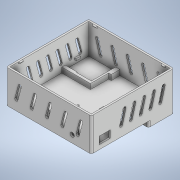
# Autodesk Inventor part: Raspberry Pi hållare 2
Saved by Autodesk Inventor 2021 (Build 250183000, 183)
## iProperties
Created: 2024-12-11
Part Number: Raspberry Pi hållare 2
Material: Generic
Document SubType Name: Modeling
Designer: 22liatho
Density: 1 g/cm^3
Appearance: Default
Author: 22liatho
Autodesk Inventor part; units mm, degrees
ref_plane "YZ Plane" through (0, 0, 0) normal (1, 0, 0) x (0, 1, 0)
ref_plane "XZ Plane" through (0, 0, 0) normal (0, 1, 0) x (-1, 0, 0)
ref_plane "XY Plane" through (0, 0, 0) normal (0, 0, 1) x (1, 0, 0)
sketch "Sketch1" plane through (0, 0, 0) normal (0, 1, 0) x (-1, 0, 0)
  line L0 (0, 0) -> (-94.1, 0)
  line L1 (-94.1, 0) -> (-94.1, -91.1)
  line L2 (-94.1, -91.1) -> (0, -91.1)
  line L3 (0, -91.1) -> (0, 0)
  line L4 (2, 2) -> (-96.1, 2)
  line L5 (-96.1, 2) -> (-96.1, -93.1)
  line L6 (-96.1, -93.1) -> (2, -93.1)
  line L7 (2, -93.1) -> (2, 2)
  dimension "d0" = 91.1
  dimension "d1" = 94.1
  dimension "d2" = 2
  dimension "d3" = 2
  dimension "d4" = 2
  dimension "d5" = 2
  constraints: 16 end point, 4 parallel, 2 horizontal, 2 perpendicular
  measures "d0" distance of L2.end L0.start
  measures "d1" distance of L1.end L2.end
  measures "d2" distance between parallel lines of L6 L2
  measures "d3" distance between parallel lines of L7 L3
  measures "d4" distance between parallel lines of L4 L0
  measures "d5" distance between parallel lines of L1 L5
extrude "Extrusion1" add sketch "Sketch1" along normal blind 2 contours L3 L2 L1 L0
extrude "Extrusion2" add sketch "Sketch1" along normal blind 38.2
sketch "Sketch3" plane through (96.1, 0, 2) normal (1, 0, 0) x (0, 0, -1)
  line L0 (12.85, 3.6) -> (19.55, 3.6)
  line L1 (19.55, 6.8) -> (12.85, 6.8)
  line L2 (11.7, 5.65) -> (11.7, 4.75)
  line L3 (20.7, 4.75) -> (20.7, 5.65)
  arc A0 (12.85, 6.8) -> (11.7, 5.65) centre (12.85, 5.65) ccw
  arc A1 (11.7, 4.75) -> (12.85, 3.6) centre (12.85, 4.75) ccw
  arc A2 (20.7, 5.65) -> (19.55, 6.8) centre (19.55, 5.65) ccw
  arc A3 (19.55, 3.6) -> (20.7, 4.75) centre (19.55, 4.75) ccw
  line L4 (0, 0) -> (0, 38.2) projected
  line L5 (0, 0) -> (95.1, 0) projected
  line L6 (12.85, 8.4) -> (19.55, 8.4)
  arc A4 (22.3, 5.65) -> (19.55, 8.4) centre (19.55, 5.65) ccw
  line L7 (22.3, 5.65) -> (22.3, 4.75)
  arc A5 (19.55, 2) -> (22.3, 4.75) centre (19.55, 4.75) ccw
  line L8 (19.55, 2) -> (12.85, 2)
  arc A6 (10.1, 4.75) -> (12.85, 2) centre (12.85, 4.75) ccw
  line L9 (10.1, 4.75) -> (10.1, 5.65)
  arc A7 (12.85, 8.4) -> (10.1, 5.65) centre (12.85, 5.65) ccw
  point P0 (2, 0)
  dimension "d15" = 1.15
  dimension "d16" = 9
  dimension "d17" = 3.2
  dimension "d18" = 11.7
  dimension "d19" = 3.6
  dimension "d22" = 1.6
  constraints: 16 end point, 16 point on circle, 8 centre point, 8 tangent, 3 equal radius, 2 horizontal, 2 perpendicular, 1 vertical, 7 other
  measures "d15" radius of A0
  measures "d16" distance between parallel lines of L2 L3
  measures "d17" distance between parallel lines of L1 L0
  measures "d18" distance between parallel lines of L4 L2
  measures "d19" distance between parallel lines of L5 L0
  measures "d22" distance between parallel lines of L1 L6
sketch "Sketch4" plane through (0, 0, 0) normal (0, -1, 0) x (1, 0, 0)
  line L0 (96.1, 2) -> (96.1, -93.1) projected
  line L1 (96.1, -93.1) -> (91.1, -93.1)
  line L2 (91.1, -93.1) -> (91.1, -68.8)
  line L3 (66.1, -63.8) -> (96.1, -63.8)
  line L4 (96.1, -63.8) -> (96.1, -93.1)
  line L5 (96.1, -93.1) -> (-2, -93.1) projected
  line L6 (71.1, -93.1) -> (66.1, -93.1)
  line L7 (66.1, -93.1) -> (66.1, -63.8)
  line L8 (71.1, -68.8) -> (71.1, -93.1)
  line L9 (71.1, -68.8) -> (91.1, -68.8)
  line L10 (93.1, -93.1) -> (93.1, -66.8)
  line L11 (93.1, -66.8) -> (69.1, -66.8)
  line L12 (69.1, -66.8) -> (69.1, -93.1)
  point P0 (0, 0)
  point P1 (96.1, -63.8)
  point P2 (66.1, -93.1)
  dimension "d25" = 5
  dimension "d26" = 5
  dimension "d28" = 26.3
  dimension "d29" = 24
  dimension "d30" = 2
  dimension "d31" = 2
  dimension "d32" = 2
  dimension "d33" = 5
  constraints: 22 end point, 4 parallel, 4 perpendicular, 3 point on line, 2 horizontal
  measures "d25" distance between parallel lines of L0 L2
  measures "d26" distance between parallel lines of L7 L8
  measures "d28" distance of L11.end L12.end
  measures "d29" distance between parallel lines of L12 L10
  measures "d30" distance between parallel lines of L12 L8
  measures "d31" distance between parallel lines of L11 L9
  measures "d32" distance between parallel lines of L10 L2
  measures "d33" distance between parallel lines of L9 L3
extrude "Extrusion6" add sketch "Sketch4" along normal blind 6.5 contours L0 L1 L10 L11 L12 L5 L7 L3 | L1 L2 L9 L8 L5 L12 L11 L10
sketch "Sketch5" plane through (96.1, 38.2, -93.1) normal (0, 0, -1) x (-1, 0, 0)
  line L0 (98.1, -38.2) -> (0, -38.2) projected
  line L1 (2.5, -38.2) -> (27.5, -38.2)
  line L2 (27.5, -38.2) -> (27.5, -43.2)
  line L3 (27.5, -43.2) -> (2.5, -43.2)
  line L4 (2.5, -43.2) -> (2.5, -38.2)
  line L5 (25, -38.2) -> (25, -44.7) projected
  line L6 (5, -38.2) -> (5, -44.7) projected
  line L7 (25, -44.7) -> (5, -44.7) projected
  point P0 (96.1, -38.2)
  dimension "d37" = 2.5
  dimension "d38" = 2.5
  dimension "d418" = 1.5
  constraints: 8 end point, 2 parallel, 1 horizontal, 1 perpendicular, 1 point on line
  measures "d37" distance between parallel lines of L5 L2
  measures "d38" distance between parallel lines of L6 L4
  measures "d418" distance between parallel lines of L7 L3
extrude "Extrusion7" cut sketch "Sketch5" against normal up to surface (24.3 mm away) contours L2 L3 L5 L0 | L5 L3 L6 L0 | L6 L3 L4 L0
sketch "Sketch6" plane through (0, 0, 0) normal (0, -1, 0) x (1, 0, 0)
  line L0 (58.6, -6.3) -> (7.5, -6.3)
  arc A0 (7.5, -6.3) -> (7.5, -9.8) centre (7.5, -8.05) ccw
  line L1 (7.5, -9.8) -> (58.6, -9.8)
  arc A1 (58.6, -9.8) -> (58.6, -6.3) centre (58.6, -8.05) ccw
  line L2 (96.1, 2) -> (96.1, -63.8) projected
  line L3 (0, 0) -> (94.1, 0) projected
  line L4 (58.6, -18.5167) -> (7.5, -18.5167)
  line L5 (7.5, -22.0167) -> (58.6, -22.0167)
  arc A2 (7.5, -18.5167) -> (7.5, -22.0167) centre (7.5, -20.2667) ccw
  arc A3 (58.6, -22.0167) -> (58.6, -18.5167) centre (58.6, -20.2667) ccw
  line L6 (58.6, -30.7333) -> (7.5, -30.7333)
  line L7 (7.5, -34.2333) -> (58.6, -34.2333)
  arc A4 (7.5, -30.7333) -> (7.5, -34.2333) centre (7.5, -32.4833) ccw
  arc A5 (58.6, -34.2333) -> (58.6, -30.7333) centre (58.6, -32.4833) ccw
  line L8 (58.6, -42.95) -> (7.5, -42.95)
  line L9 (7.5, -46.45) -> (58.6, -46.45)
  arc A6 (7.5, -42.95) -> (7.5, -46.45) centre (7.5, -44.7) ccw
  arc A7 (58.6, -46.45) -> (58.6, -42.95) centre (58.6, -44.7) ccw
  line L10 (58.6, -55.1667) -> (7.5, -55.1667)
  line L11 (7.5, -58.6667) -> (58.6, -58.6667)
  arc A8 (7.5, -55.1667) -> (7.5, -58.6667) centre (7.5, -56.9167) ccw
  arc A9 (58.6, -58.6667) -> (58.6, -55.1667) centre (58.6, -56.9167) ccw
  line L12 (58.6, -67.3833) -> (7.5, -67.3833)
  line L13 (7.5, -70.8833) -> (58.6, -70.8833)
  arc A10 (7.5, -67.3833) -> (7.5, -70.8833) centre (7.5, -69.1333) ccw
  arc A11 (58.6, -70.8833) -> (58.6, -67.3833) centre (58.6, -69.1333) ccw
  line L14 (58.6, -79.6) -> (7.5, -79.6)
  line L15 (7.5, -83.1) -> (58.6, -83.1)
  arc A12 (7.5, -79.6) -> (7.5, -83.1) centre (7.5, -81.35) ccw
  arc A13 (58.6, -83.1) -> (58.6, -79.6) centre (58.6, -81.35) ccw
  line L16 (66.1, -93.1) -> (-2, -93.1) projected
  line L17 (66.1, -63.8) -> (66.1, -93.1) projected
  arc A14 (106.65, -9.8) -> (106.65, -6.3) centre (106.65, -8.05) ccw
  line L18 (106.65, -6.3) -> (55.55, -6.3)
  line L19 (55.55, -9.8) -> (106.65, -9.8)
  arc A15 (55.55, -6.3) -> (55.55, -9.8) centre (55.55, -8.05) ccw
  line L20 (55.55, -22.3) -> (106.65, -22.3)
  arc A16 (106.65, -22.3) -> (106.65, -18.8) centre (106.65, -20.55) ccw
  line L21 (106.65, -18.8) -> (55.55, -18.8)
  arc A17 (55.55, -18.8) -> (55.55, -22.3) centre (55.55, -20.55) ccw
  line L22 (55.55, -34.8) -> (106.65, -34.8)
  arc A18 (106.65, -34.8) -> (106.65, -31.3) centre (106.65, -33.05) ccw
  line L23 (106.65, -31.3) -> (55.55, -31.3)
  arc A19 (55.55, -31.3) -> (55.55, -34.8) centre (55.55, -33.05) ccw
  line L24 (55.55, -47.3) -> (106.65, -47.3)
  arc A20 (106.65, -47.3) -> (106.65, -43.8) centre (106.65, -45.55) ccw
  line L25 (106.65, -43.8) -> (55.55, -43.8)
  arc A21 (55.55, -43.8) -> (55.55, -47.3) centre (55.55, -45.55) ccw
  line L26 (55.55, -59.8) -> (106.65, -59.8)
  arc A22 (106.65, -59.8) -> (106.65, -56.3) centre (106.65, -58.05) ccw
  line L27 (106.65, -56.3) -> (55.55, -56.3)
  arc A23 (55.55, -56.3) -> (55.55, -59.8) centre (55.55, -58.05) ccw
  line L28 (55.55, -72.3) -> (106.65, -72.3)
  arc A24 (106.65, -72.3) -> (106.65, -68.8) centre (106.65, -70.55) ccw
  line L29 (106.65, -68.8) -> (55.55, -68.8)
  arc A25 (55.55, -68.8) -> (55.55, -72.3) centre (55.55, -70.55) ccw
  line L30 (55.55, -84.8) -> (106.65, -84.8)
  arc A26 (106.65, -84.8) -> (106.65, -81.3) centre (106.65, -83.05) ccw
  line L31 (106.65, -81.3) -> (55.55, -81.3)
  arc A27 (55.55, -81.3) -> (55.55, -84.8) centre (55.55, -83.05) ccw
  line L32 (71.1, -68.8) -> (91.1, -68.8) projected
  line L33 (91.1, -68.8) -> (91.1, -93.1) projected
  line L34 (71.1, -93.1) -> (71.1, -68.8) projected
  line L35 (96.1, -63.8) -> (66.1, -63.8) projected
  line L36 (91.1, -93.1) -> (-2, -93.1) projected
  line L37 (-2, 2) -> (96.1, 2) projected
  point P0 (93.6, -93.1)
  point P1 (68.6, -93.1)
  point P2 (96.1, -93.1)
  dimension "d42" = 7.5
  dimension "d43" = 3.5
  dimension "d47" = 12.2167
  dimension "d52" = 10
  dimension "d53" = 7.5
  dimension "d56" = 48.05
  dimension "d64" = 12.5
  dimension "d70" = 15.55
  dimension "d71" = 15.55
  dimension "d74" = 8.3
  dimension "d75" = 8.3
  constraints: 56 end point, 56 point on circle, 28 centre point, 4 tangent, 3 horizontal, 2 vertical, 1 point on line, 130 other
  measures "d42" horizontal distance of L3.start L1.start
  measures "d43" distance between parallel lines of L1 L0
  measures "d47" distance of L0.start L4.start
  measures "d52" distance between parallel lines of L16 L15
  measures "d53" distance from line of A13.centre L17
  measures "d56" distance of A1.centre A14.centre
  measures "d64" distance of L19.start L20.start
  measures "d70" distance from line of L33 A24.centre
  measures "d71" distance from line of L34 A27.centre
  measures "d74" distance between parallel lines of L37 L18
  measures "d75" distance between parallel lines of L36 L30
sketch "Sketch7" plane through (0, 0, 0) normal (0, -1, 0) x (1, 0, 0)
  line L0 (83.6, -43.799) -> (10.5, -43.799)
  arc A0 (83.6, -47.299) -> (83.6, -43.799) centre (83.6, -45.549) ccw
  line L1 (83.6, -47.299) -> (10.5, -47.299)
  arc A1 (10.5, -43.799) -> (10.5, -47.299) centre (10.5, -45.549) ccw
  line L2 (96.1, 2) -> (96.1, -63.8) projected
  line L3 (91.1, -68.8) -> (91.1, -93.1) projected
  line L4 (71.1, -93.1) -> (71.1, -68.8) projected
  line L5 (-2, -93.1) -> (-2, 2) projected
  line L6 (83.6, -59.2327) -> (10.5, -59.2327)
  arc A2 (10.5, -55.7327) -> (10.5, -59.2327) centre (10.5, -57.4827) ccw
  line L7 (83.6, -55.7327) -> (10.5, -55.7327)
  arc A3 (83.6, -59.2327) -> (83.6, -55.7327) centre (83.6, -57.4827) ccw
  line L8 (56.1, -67.6663) -> (10.5, -67.6663)
  arc A4 (10.5, -67.6663) -> (10.5, -71.1663) centre (10.5, -69.4163) ccw
  line L9 (10.5, -71.1663) -> (56.1, -71.1663)
  arc A5 (56.1, -71.1663) -> (56.1, -67.6663) centre (56.1, -69.4163) ccw
  line L10 (-2, 2) -> (96.1, 2) projected
  line L11 (96.1, -63.8) -> (66.1, -63.8) projected
  line L12 (66.1, -63.8) -> (66.1, -93.1) projected
  line L13 (10.5, -83.1) -> (56.1, -83.1)
  arc A6 (10.5, -79.6) -> (10.5, -83.1) centre (10.5, -81.35) ccw
  line L14 (56.1, -79.6) -> (10.5, -79.6)
  arc A7 (56.1, -83.1) -> (56.1, -79.6) centre (56.1, -81.35) ccw
  line L15 (66.1, -93.1) -> (-2, -93.1) projected
  line L16 (83.6, -19.9317) -> (38, -19.9317)
  arc A8 (38, -19.9317) -> (38, -23.4317) centre (38, -21.6817) ccw
  line L17 (38, -23.4317) -> (83.6, -23.4317)
  arc A9 (83.6, -23.4317) -> (83.6, -19.9317) centre (83.6, -21.6817) ccw
  arc A10 (38, -7.9977) -> (38, -11.4977) centre (38, -9.7477) ccw
  line L18 (38, -11.4977) -> (83.6, -11.4977)
  arc A11 (83.6, -11.4977) -> (83.6, -7.9977) centre (83.6, -9.7477) ccw
  line L19 (83.6, -7.9977) -> (38, -7.9977)
  line L20 (83.6, -31.8653) -> (10.5, -31.8653)
  arc A12 (83.6, -35.3653) -> (83.6, -31.8653) centre (83.6, -33.6153) ccw
  arc A13 (10.5, -31.8653) -> (10.5, -35.3653) centre (10.5, -33.6153) ccw
  line L21 (83.6, -35.3653) -> (10.5, -35.3653)
  point P0 (0, 0)
  point P1 (96.1, -93.1)
  dimension "d76" = 3.5
  dimension "d80" = 12.5
  dimension "d81" = 12.5
  dimension "d84" = 11.9337
  dimension "d89" = 45.799
  dimension "d92" = 10
  dimension "d93" = 3.5
  dimension "d96" = 11.9337
  dimension "d102" = 10
  dimension "d391" = 11.9337
  dimension "d392" = 12.5
  dimension "d393" = 3.5
  dimension "d394" = 12.5
  dimension "d395" = 45.6
  dimension "d396" = 45.6
  dimension "d397" = 23.8673
  dimension "d400" = 11.934
  dimension "d411" = 11.9337
  constraints: 28 end point, 28 point on circle, 14 centre point, 12 tangent, 6 horizontal, 4 vertical, 40 other
  measures "d76" distance between parallel lines of L0 L1
  measures "d80" distance from line of L5 A1.centre
  measures "d81" distance from line of L2 A0.centre
  measures "d84" distance of L1.start L6.start
  measures "d89" distance between parallel lines of L10 L0
  measures "d92" distance from line of L12 A5.centre
  measures "d93" distance between parallel lines of L9 L8
  measures "d96" distance of L9.start L13.start
  measures "d102" distance between parallel lines of L15 L13
  measures "d391" distance between parallel lines of L9 L6
  measures "d392" distance from line of L5 A6.centre
  measures "d393" distance between parallel lines of L17 L16
  measures "d394" distance from line of L2 A9.centre
  measures "d395" distance of L8.start L8.end
  measures "d396" distance of L16.start L16.end
  measures "d397" distance between parallel lines of L0 L16
  measures "d400" distance of L17.start L18.start
  measures "d411" distance of L0.start L20.start
extrude "Extrusion8" [suppressed]
sketch "Sketch10" plane through (-2, 0, 2) normal (0, 0, 1) x (1, 0, 0)
  arc A0 (17.4, 26.1471) -> (14.0192, 27.0529) centre (15.7096, 26.6) ccw
  arc A1 (10, 12.0529) -> (13.3807, 11.1471) centre (11.6904, 11.6) ccw
  line L0 (13.3807, 11.1471) -> (17.4, 26.1471)
  line L1 (10, 12.0529) -> (14.0192, 27.0529)
  line L2 (0, 38.2) -> (98.1, 38.2)
  line L3 (13.3807, 11.1471) -> (14.3807, 11.1471)
  line L4 (14.3807, 11.1471) -> (13.8807, 11.1471)
  line L5 (98.1, 0) -> (98.1, 38.2) projected
  line L6 (0, 0) -> (98.1, 0) projected
  line L7 (0, 0) -> (0, 38.2) projected
  arc A2 (27.675, 12.0529) -> (31.0557, 11.1471) centre (29.3654, 11.6) ccw
  line L8 (27.675, 12.0529) -> (31.6942, 27.0529)
  line L9 (32.0557, 11.1471) -> (31.5557, 11.1471)
  line L10 (31.0557, 11.1471) -> (35.075, 26.1471)
  arc A3 (35.075, 26.1471) -> (31.6942, 27.0529) centre (33.3846, 26.6) ccw
  line L11 (31.0557, 11.1471) -> (32.0557, 11.1471)
  arc A4 (45.35, 12.0529) -> (48.7308, 11.1471) centre (47.0404, 11.6) ccw
  line L12 (45.35, 12.0529) -> (49.3692, 27.0529)
  line L13 (49.7308, 11.1471) -> (49.2308, 11.1471)
  line L14 (48.7308, 11.1471) -> (52.75, 26.1471)
  arc A5 (52.75, 26.1471) -> (49.3692, 27.0529) centre (51.0596, 26.6) ccw
  line L15 (48.7308, 11.1471) -> (49.7308, 11.1471)
  arc A6 (63.025, 12.0529) -> (66.4058, 11.1471) centre (64.7154, 11.6) ccw
  line L16 (63.025, 12.0529) -> (67.0443, 27.0529)
  line L17 (67.4058, 11.1471) -> (66.9058, 11.1471)
  line L18 (66.4058, 11.1471) -> (70.425, 26.1471)
  arc A7 (70.425, 26.1471) -> (67.0443, 27.0529) centre (68.7346, 26.6) ccw
  line L19 (66.4058, 11.1471) -> (67.4058, 11.1471)
  arc A8 (80.7, 12.0529) -> (84.0808, 11.1471) centre (82.3904, 11.6) ccw
  line L20 (80.7, 12.0529) -> (84.7193, 27.0529)
  line L21 (85.0808, 11.1471) -> (84.5808, 11.1471)
  line L22 (84.0808, 11.1471) -> (88.1, 26.1471)
  arc A9 (88.1, 26.1471) -> (84.7193, 27.0529) centre (86.4096, 26.6) ccw
  line L23 (84.0808, 11.1471) -> (85.0808, 11.1471)
  dimension "d133" = 3.5
  dimension "d134" = 15
  dimension "d137" = 75
  dimension "d138" = 1
  dimension "d145" = 10
  dimension "d364" = 11.6
  dimension "d365" = 11.6
  dimension "d368" = 17.675
  dimension "d376" = 10
  constraints: 42 end point, 20 point on circle, 10 centre point, 4 tangent, 3 horizontal, 1 midpoint, 1 parallel, 56 other
  measures "d133" distance between parallel lines of L1 L0
  measures "d134" vertical distance of A1.centre A0.centre
  measures "d137" angle of L0 L3
  measures "d138" distance of L0.start L4.start
  measures "d145" distance from line of L7 L1.start
  measures "d364" distance from line of L6 A1.centre
  measures "d365" distance from line of L2 A0.centre
  measures "d368" distance of L1.start L8.start
  measures "d376" distance from line of L5 L22.end
sketch "Sketch9" plane through (-2, 0, 2) normal (0, 0, 1) x (1, 0, 0)
  line L0 (73.6, 6) -> (78.6, 6)
  line L1 (78.6, 6) -> (78.6, 11)
  line L2 (78.6, 11) -> (73.6, 11)
  line L3 (73.6, 11) -> (73.6, 6)
  line L4 (0, 0) -> (98.1, 0) projected
  line L5 (98.1, 0) -> (98.1, 38.2) projected
  circle A0 centre (76.1, 8.5) radius 2.5
  point P0 (2, 0)
  dimension "d126" = 5
  dimension "d127" = 19.5
  dimension "d128" = 5
  dimension "d380" = 5
  dimension "d475" = 8.5
  constraints: 8 end point, 2 parallel, 2 tangent, 1 centre point, 1 horizontal, 1 perpendicular
  measures "d126" distance between parallel lines of L3 L1
  measures "d127" distance between parallel lines of L5 L1
  measures "d128" distance between parallel lines of L0 L2
  measures "d380" diameter of A0
  measures "d475" distance from line of L4 A0.centre
extrude "Extrusion10" cut sketch "Sketch10" against normal blind 10 contours L0 A1 L1 A0
sketch "Sketch12" plane through (0, 2, -91.1) normal (0, 0, 1) x (1, 0, 0)
  line L0 (96.1, 36.2) -> (-2, 36.2) projected
  line L1 (5, 36.2) -> (10, 36.2)
  line L2 (10, 36.2) -> (10, 34.2)
  line L3 (10, 34.2) -> (5, 34.2)
  line L4 (5, 34.2) -> (5, 36.2)
  line L5 (84.1, 36.2) -> (89.1, 36.2)
  line L6 (89.1, 36.2) -> (89.1, 34.2)
  line L7 (89.1, 34.2) -> (84.1, 34.2)
  line L8 (84.1, 34.2) -> (84.1, 36.2)
  line L9 (0, 0) -> (0, 36.2) projected
  line L10 (94.1, 0) -> (94.1, 36.2) projected
  point P0 (0, -2)
  point P1 (-2, 36.2)
  point P2 (58.1, 29.2)
  dimension "d170" = 5
  dimension "d171" = 2
  dimension "d172" = 5
  dimension "d173" = 5
  dimension "d536" = 5
  constraints: 16 end point, 4 parallel, 2 horizontal, 2 perpendicular, 1 point on line, 3 other
  measures "d170" distance of L2.end L3.end
  measures "d171" distance of L1.end L2.end
  measures "d172" distance of L6.end L7.end
  measures "d173" distance between parallel lines of L9 L4
  measures "d536" distance from line of L10 L5.end
extrude "Extrusion11" add sketch "Sketch12" along normal blind 1.4
sketch "Sketch13" plane through (0, 2, -91.1) normal (1, 0, 0) x (0, 0, -1)
  line L0 (2, 36.2) -> (-93.1, 36.2) projected
  line L1 (-81.1, 36.2) -> (-76.1, 36.2)
  line L2 (-76.1, 36.2) -> (-76.1, 34.2)
  line L3 (-76.1, 34.2) -> (-81.1, 34.2)
  line L4 (-81.1, 34.2) -> (-81.1, 36.2)
  line L5 (-91.1, 0) -> (-91.1, 36.2) projected
  point P0 (-91.1, -2)
  point P1 (-76.1, 36.2)
  dimension "d201" = 2
  dimension "d202" = 5
  dimension "d203" = 10
  constraints: 8 end point, 2 parallel, 1 horizontal, 1 perpendicular, 1 point on line
  measures "d201" distance of L1.end L2.end
  measures "d202" distance of L2.end L3.end
  measures "d203" distance between parallel lines of L5 L4
extrude "Extrusion12" add sketch "Sketch13" along normal blind 1.4
chamfer "Chamfer9" distance 0.75 distance2 1.4 1 edges at (1.4, 38.2, -12.5) measured on face at (1.4, 37.5333, -11.6667)
chamfer "Chamfer10" distance 0.75 distance2 1.4 1 edges at (1.4, 36.825, -10) measured on face at (1.4, 37.0333, -11.6667)
chamfer "Chamfer11" distance 0.75 distance2 1.4 1 edges at (1.4, 36.825, -15) measured on face at (1.4, 37.0333, -12.1666)
chamfer "Chamfer12" distance 0.75 distance2 1.4 1 edges at (1.4, 36.2, -12.5) measured on face at (1.4, 37.0333, -11.9166)
sketch "Sketch14" plane through (94.1, 2, -91.1) normal (-1, 0, 0) x (0, 0, 1)
  line L0 (93.1, 36.2) -> (-2, 36.2) projected
  line L1 (81.1, 36.2) -> (76.1, 36.2)
  line L2 (76.1, 36.2) -> (76.1, 34.2)
  line L3 (76.1, 34.2) -> (81.1, 34.2)
  line L4 (81.1, 34.2) -> (81.1, 36.2)
  line L5 (93.1, -2) -> (93.1, 36.2) projected
  line L6 (91.1, 0) -> (91.1, 36.2) projected
  point P0 (91.1, -2)
  dimension "d242" = 5
  dimension "d243" = 2
  dimension "d537" = 10
  constraints: 8 end point, 2 parallel, 1 horizontal, 1 perpendicular, 1 point on line
  measures "d242" distance of L2.end L3.end
  measures "d243" distance of L3.end L1.start
  measures "d537" distance between parallel lines of L6 L4
extrude "Extrusion13" add sketch "Sketch14" along normal blind 1.4
chamfer "Chamfer25" distance 0.75 distance2 1.4 1 edges at (10, 37.2, -89.7) measured on face at (8.3333, 36.8667, -89.7)
chamfer "Chamfer26" distance 0.75 distance2 1.4 1 edges at (5, 37.2, -89.7) measured on face at (6.4167, 36.8667, -89.7)
chamfer "Chamfer27" distance 0.75 distance2 1.4 2 edges at (7.5, 38.2, -89.7) (86.6, 38.2, -89.7) measured on face at (87.4333, 36.8667, -89.7) measured on face at (6.9166, 36.8667, -89.7)
chamfer "Chamfer28" distance 0.75 distance2 1.4 1 edges at (7.5, 36.2, -89.7) measured on face at (6.9166, 36.6167, -89.7)
chamfer_without_effect "Chamfer29"
chamfer "Chamfer30" distance 0.75 distance2 1.4 1 edges at (84.1, 36.825, -89.7) measured on face at (85.7667, 37.0333, -89.7)
chamfer "Chamfer31" distance 0.75 distance2 1.4 1 edges at (86.9749, 36.2, -89.7) measured on face at (86.2666, 37.0333, -89.7)
chamfer "Chamfer32" distance 0.75 distance2 1.4 1 edges at (89.1, 37.2, -89.7) measured on face at (86.2666, 37.2833, -89.7)
chamfer "Chamfer33" distance 0.75 distance2 1.4 1 edges at (92.7, 37.2, -10) measured on face at (92.7, 36.8667, -11.6667)
chamfer "Chamfer34" distance 0.75 distance2 1.4 1 edges at (92.7, 37.2, -15) measured on face at (92.7, 36.8667, -12.1666)
chamfer "Chamfer35" distance 0.75 distance2 1.4 1 edges at (92.7, 38.2, -12.5) measured on face at (92.7, 36.8667, -11.9166)
chamfer "Chamfer36" distance 0.75 distance2 1.4 1 edges at (92.7, 36.2, -12.5) measured on face at (92.7, 36.6167, -11.9166)
sketch "Sketch16" plane through (96.1, 38.2, -93.1) normal (0, 0, -1) x (-1, 0, 0)
  line L0 (10, -26.6) -> (14.0192, -11.6)
  arc A0 (10, -26.6) -> (13.3807, -27.5059) centre (11.6904, -27.0529) ccw
  line L1 (14.3807, -27.5059) -> (13.8807, -27.5059)
  line L2 (13.3807, -27.5059) -> (17.4, -12.5059)
  line L3 (13.3807, -27.5059) -> (14.3807, -27.5059)
  arc A1 (17.4, -12.5059) -> (14.0192, -11.6) centre (15.7096, -12.0529) ccw
  line L4 (98.1, -38.2) -> (98.1, 0) projected
  line L5 (0, -44.7) -> (0, 0) projected
  line L6 (0, 0) -> (98.1, 0) projected
  arc A2 (27.675, -26.6) -> (31.0557, -27.5059) centre (29.3654, -27.0529) ccw
  line L7 (27.675, -26.6) -> (31.6942, -11.6)
  line L8 (32.0557, -27.5059) -> (31.5557, -27.5059)
  line L9 (31.0557, -27.5059) -> (32.0557, -27.5059)
  line L10 (31.0557, -27.5059) -> (35.075, -12.5059)
  arc A3 (35.075, -12.5059) -> (31.6942, -11.6) centre (33.3846, -12.0529) ccw
  arc A4 (45.35, -26.6) -> (48.7308, -27.5059) centre (47.0404, -27.0529) ccw
  line L11 (45.35, -26.6) -> (49.3692, -11.6)
  line L12 (49.7308, -27.5059) -> (49.2308, -27.5059)
  line L13 (48.7308, -27.5059) -> (49.7308, -27.5059)
  line L14 (48.7308, -27.5059) -> (52.75, -12.5059)
  arc A5 (52.75, -12.5059) -> (49.3692, -11.6) centre (51.0596, -12.0529) ccw
  arc A6 (63.025, -26.6) -> (66.4058, -27.5059) centre (64.7154, -27.0529) ccw
  line L15 (63.025, -26.6) -> (67.0443, -11.6)
  line L16 (67.4058, -27.5059) -> (66.9058, -27.5059)
  line L17 (66.4058, -27.5059) -> (67.4058, -27.5059)
  line L18 (66.4058, -27.5059) -> (70.425, -12.5059)
  arc A7 (70.425, -12.5059) -> (67.0443, -11.6) centre (68.7346, -12.0529) ccw
  arc A8 (80.7, -26.6) -> (84.0808, -27.5059) centre (82.3904, -27.0529) ccw
  line L19 (80.7, -26.6) -> (84.7193, -11.6)
  line L20 (85.0808, -27.5059) -> (84.5808, -27.5059)
  line L21 (84.0808, -27.5059) -> (85.0808, -27.5059)
  line L22 (84.0808, -27.5059) -> (88.1, -12.5059)
  arc A9 (88.1, -12.5059) -> (84.7193, -11.6) centre (86.4096, -12.0529) ccw
  point P0 (96.1, -38.2)
  point P1 (98.1, -19.1)
  point P2 (12.0096, -19.1)
  point P3 (29.6846, -19.1)
  point P4 (47.3596, -19.1)
  point P5 (65.0346, -19.1)
  point P6 (82.7096, -19.1)
  point P7 (98.1, -19.1)
  point P8 (0, -38.2)
  dimension "d327" = 3.5
  dimension "d328" = 15
  dimension "d329" = 75
  dimension "d330" = 1
  dimension "d336" = 17.675
  dimension "d377" = 10
  dimension "d378" = 10
  constraints: 40 end point, 20 point on circle, 10 centre point, 4 midpoint, 4 tangent, 2 horizontal, 1 horizontal alignment, 1 parallel, 60 other
  measures "d327" distance between parallel lines of L0 L2
  measures "d328" vertical distance of A0.centre A1.centre
  measures "d329" angle of L2 L3
  measures "d330" distance of L3.start L1.start
  measures "d336" distance of A0.centre A2.centre
  measures "d377" distance from line of L4 L22.end
  measures "d378" distance from line of L5 L0.start
extrude "Extrusion16" cut sketch "Sketch16" against normal blind 2
sketch "Sketch19" plane through (96.1, 0, 2) normal (1, 0, 0) x (0, 0, -1)
  arc A0 (77.7, 12.0529) -> (81.0808, 11.1471) centre (79.3904, 11.6) ccw
  line L0 (77.7, 12.0529) -> (81.7193, 27.0529)
  line L1 (82.0808, 11.1471) -> (81.5808, 11.1471)
  line L2 (81.0808, 11.1471) -> (82.0808, 11.1471)
  line L3 (81.0808, 11.1471) -> (85.1, 26.1471)
  arc A1 (85.1, 26.1471) -> (81.7193, 27.0529) centre (83.4096, 26.6) ccw
  line L4 (95.1, -6.5) -> (95.1, 38.2) projected
  line L5 (95.1, 11.6) -> (95.1, 26.6) projected
  line L6 (0, 38.2) -> (95.1, 38.2) projected
  arc A2 (73.8167, 26.1471) -> (70.4359, 27.0529) centre (72.1263, 26.6) ccw
  line L7 (69.7974, 11.1471) -> (73.8167, 26.1471)
  line L8 (70.7974, 11.1471) -> (70.2974, 11.1471)
  line L9 (69.7974, 11.1471) -> (70.7974, 11.1471)
  line L10 (66.4167, 12.0529) -> (70.4359, 27.0529)
  arc A3 (66.4167, 12.0529) -> (69.7974, 11.1471) centre (68.1071, 11.6) ccw
  arc A4 (62.5333, 26.1471) -> (59.1526, 27.0529) centre (60.843, 26.6) ccw
  line L11 (58.5141, 11.1471) -> (62.5333, 26.1471)
  line L12 (59.5141, 11.1471) -> (59.0141, 11.1471)
  line L13 (58.5141, 11.1471) -> (59.5141, 11.1471)
  line L14 (55.1333, 12.0529) -> (59.1526, 27.0529)
  arc A5 (55.1333, 12.0529) -> (58.5141, 11.1471) centre (56.8237, 11.6) ccw
  arc A6 (51.25, 26.1471) -> (47.8692, 27.0529) centre (49.5596, 26.6) ccw
  line L15 (47.2308, 11.1471) -> (51.25, 26.1471)
  line L16 (48.2308, 11.1471) -> (47.7308, 11.1471)
  line L17 (47.2308, 11.1471) -> (48.2308, 11.1471)
  line L18 (43.85, 12.0529) -> (47.8692, 27.0529)
  arc A7 (43.85, 12.0529) -> (47.2308, 11.1471) centre (45.5404, 11.6) ccw
  arc A8 (39.9667, 26.1471) -> (36.5859, 27.0529) centre (38.2763, 26.6) ccw
  line L19 (35.9474, 11.1471) -> (39.9667, 26.1471)
  line L20 (36.9474, 11.1471) -> (36.4474, 11.1471)
  line L21 (35.9474, 11.1471) -> (36.9474, 11.1471)
  line L22 (32.5667, 12.0529) -> (36.5859, 27.0529)
  arc A9 (32.5667, 12.0529) -> (35.9474, 11.1471) centre (34.257, 11.6) ccw
  arc A10 (28.6833, 26.1471) -> (25.3026, 27.0529) centre (26.9929, 26.6) ccw
  line L23 (24.6641, 11.1471) -> (28.6833, 26.1471)
  line L24 (25.6641, 11.1471) -> (25.1641, 11.1471)
  line L25 (24.6641, 11.1471) -> (25.6641, 11.1471)
  line L26 (21.2833, 12.0529) -> (25.3026, 27.0529)
  arc A11 (21.2833, 12.0529) -> (24.6641, 11.1471) centre (22.9737, 11.6) ccw
  arc A12 (17.4, 26.1471) -> (14.0192, 27.0529) centre (15.7096, 26.6) ccw
  line L27 (13.3807, 11.1471) -> (17.4, 26.1471)
  line L28 (14.3807, 11.1471) -> (13.8807, 11.1471)
  line L29 (13.3807, 11.1471) -> (14.3807, 11.1471)
  line L30 (10, 12.0529) -> (14.0192, 27.0529)
  arc A13 (10, 12.0529) -> (13.3807, 11.1471) centre (11.6904, 11.6) ccw
  line L31 (0, 0) -> (0, 38.2) projected
  point P0 (2, 0)
  point P1 (79.7096, 19.5529)
  point P2 (95.1, 19.1)
  point P3 (83.0904, 18.6471)
  point P4 (71.807, 18.6471)
  point P5 (68.4263, 19.5529)
  point P6 (60.5237, 18.6471)
  point P7 (57.143, 19.5529)
  point P8 (49.2404, 18.6471)
  point P9 (45.8596, 19.5529)
  point P10 (37.957, 18.6471)
  point P11 (34.5763, 19.5529)
  point P12 (26.6737, 18.6471)
  point P13 (23.293, 19.5529)
  point P14 (15.3904, 18.6471)
  point P15 (12.0096, 19.5529)
  point P16 (95.1, 0)
  dimension "d348" = 3.5
  dimension "d349" = 15
  dimension "d350" = 75
  dimension "d351" = 1
  dimension "d357" = 11.2833
  dimension "d379" = 10
  dimension "d427" = 10
  dimension "d525" = 11.6
  constraints: 56 end point, 28 point on circle, 14 centre point, 4 midpoint, 4 tangent, 2 horizontal, 1 parallel, 96 other
  measures "d348" distance between parallel lines of L0 L3
  measures "d349" vertical distance of A0.centre A1.centre
  measures "d350" angle of L3 L2
  measures "d351" distance of L3.start L1.start
  measures "d357" distance of L3.end L7.end
  measures "d379" distance from line of L4 L3.end
  measures "d427" distance from line of L31 L30.start
  measures "d525" distance from line of L6 A1.centre
extrude "Extrusion19" cut sketch "Sketch19" against normal blind 50 contours L0 A1 L3 A0 | L7 A3 L10 A2 | L11 A5 L14 A4 | L15 A7 L18 A6 | L19 A9 L22 A8
extrude "Extrusion20" cut sketch "Sketch10" against normal blind 50 contours L8 A3 L10 A2 | L12 A5 L14 A4 | L16 A7 L18 A6 | L20 A9 L22 A8
extrude "Extrusion21" cut sketch "Sketch9" against normal blind 10 contours A0
extrude "Extrusion25" [suppressed]
extrude "Extrusion26" [suppressed]
sketch "Sketch22" plane through (0, -6.5, 0) normal (0, -1, 0) x (1, 0, 0)
  line L0 (71.1, -68.8) -> (91.1, -68.8) projected
  line L1 (96.1, -63.8) -> (66.1, -63.8) projected
  line L2 (89.1, -68.8) -> (73.1, -68.8)
  line L3 (73.1, -68.8) -> (73.1, -63.8)
  line L4 (73.1, -63.8) -> (89.1, -63.8)
  line L5 (89.1, -63.8) -> (89.1, -68.8)
  point P0 (0, 0)
  point P1 (81.1, -68.8)
  point P2 (81.1, -68.8)
  point P3 (81.1, -68.8)
  point P4 (89.1, -63.8)
  point P5 (73.1, -68.8)
  dimension "d419" = 16
  constraints: 8 end point, 3 midpoint, 2 coincident, 2 parallel, 2 point on line, 1 horizontal, 1 perpendicular
  measures "d419" distance between parallel lines of L5 L3
extrude "Extrusion27" cut sketch "Sketch22" against normal up to surface (6.5 mm away)
sketch "Sketch25" plane through (0, 2, 0) normal (0, 1, 0) x (1, 0, 0)
  line L0 (36, 0) -> (33, 0)
  line L1 (33, 0) -> (33, 10)
  line L2 (33, 10) -> (36, 10)
  line L3 (36, 10) -> (36, 0)
  line L4 (0, 0) -> (0, 91.1) projected
  line L5 (94.1, 0) -> (0, 0) projected
  point P0 (0, 10)
  dimension "d461" = 33
  dimension "d462" = 3
  dimension "d463" = 10
  constraints: 8 end point, 2 parallel, 1 horizontal, 1 perpendicular, 1 point on line
  measures "d461" distance between parallel lines of L4 L1
  measures "d462" distance between parallel lines of L3 L1
  measures "d463" distance of L2.end L0.start
extrude "Extrusion31" add sketch "Sketch25" along normal blind 6
sketch "Sketch26" plane through (0, 2, 0) normal (0, 1, 0) x (1, 0, 0)
  line L0 (94.1, 91.1) -> (0, 91.1) projected
  line L1 (36, 91.1) -> (33, 91.1)
  line L2 (33, 91.1) -> (33, 81.1)
  line L3 (33, 81.1) -> (36, 81.1)
  line L4 (36, 81.1) -> (36, 91.1)
  line L5 (0, 0) -> (0, 91.1) projected
  point P0 (0, 15)
  dimension "d466" = 3
  dimension "d467" = 33
  dimension "d528" = 10
  constraints: 8 end point, 2 parallel, 1 horizontal, 1 perpendicular, 1 point on line
  measures "d466" distance between parallel lines of L4 L2
  measures "d467" distance between parallel lines of L5 L2
  measures "d528" distance between parallel lines of L0 L3
extrude "Extrusion32" add sketch "Sketch26" along normal blind 6
sketch "Sketch27" plane through (0, 0, 0) normal (0, -1, 0) x (1, 0, 0)
  line L0 (68.6, -93.1) -> (68.6, -68.8) projected
  line L1 (93.6, -93.1) -> (-2, -93.1) projected
  line L2 (68.6, -90.1) -> (69.6, -90.1)
  line L3 (69.6, -90.1) -> (69.6, -93.1)
  line L4 (69.6, -93.1) -> (68.6, -93.1)
  line L5 (68.6, -93.1) -> (68.6, -90.1)
  line L6 (94.1, -91.1) -> (36, -91.1) projected
  line L7 (93.6, -93.1) -> (92.6, -93.1)
  line L8 (92.6, -93.1) -> (92.6, -91.1)
  line L9 (92.6, -91.1) -> (93.6, -91.1)
  line L10 (93.6, -91.1) -> (93.6, -93.1)
  point P0 (0, 0)
  point P1 (68.6, -69.3)
  point P2 (36, -91.1)
  point P3 (96.1, -93.1)
  dimension "d476" = 3
  dimension "d477" = 1
  dimension "d480" = 1
  constraints: 16 end point, 4 parallel, 2 horizontal, 2 perpendicular, 2 point on line, 2 other
  measures "d476" distance of L2.end L3.end
  measures "d477" distance between parallel lines of L0 L3
  measures "d480" distance between parallel lines of L10 L8
extrude "Extrusion34" add sketch "Sketch27" along normal blind 3.9 contours L0 L6 L3 L1 | L0 L2 L3 L6
extrude "Extrusion35" add sketch "Sketch27" along normal blind 3.9 contours L8 L6 L10 L1
sketch "Sketch28" plane through (0, 2, 0) normal (0, 1, 0) x (1, 0, 0)
  line L0 (0, 0) -> (0, 91.1) projected
  line L1 (0, 91.1) -> (5, 91.1) projected
  line L2 (0, 91.1) -> (5, 91.1) projected
  line L3 (31, 63.1) -> (31, 91.1)
  line L4 (31, 91.1) -> (33, 91.1)
  line L5 (33, 91.1) -> (33, 60.1)
  line L6 (31, 63.1) -> (14, 63.1)
  line L7 (14, 60.1) -> (33, 60.1)
  line L8 (0, 91.1) -> (0, 0) projected
  line L9 (0, 63.9) -> (14, 63.9)
  line L10 (14, 63.9) -> (14, 63.1)
  line L11 (14, 60.1) -> (0, 60.1)
  line L12 (0, 60.1) -> (0, 63.9)
  point P0 (0, 15)
  point P1 (10, 91.1)
  point P2 (84.1, 91.1)
  point P3 (0, 60.1)
  point P4 (0, 63.9)
  dimension "d586" = 31
  dimension "d587" = 2
  dimension "d588" = 3
  dimension "d589" = 28
  dimension "d592" = 14
  dimension "d594" = 27.2
  dimension "d600" = 14
  dimension "d602" = 33
  dimension "d604" = 0
  dimension "d606" = 0
  dimension "d635" = 90
  dimension "d636" = 0
  dimension "d637" = 27.2
  dimension "d638" = 30
  constraints: 19 end point, 3 parallel, 2 horizontal, 2 point on line, 1 perpendicular
  measures "d586" distance between parallel lines of L0 L3
  measures "d587" distance between parallel lines of L5 L3
  measures "d588" distance between parallel lines of L6 L7
  measures "d589" distance between parallel lines of L2 L6
  measures "d592" distance of L7.start L11.end
  measures "d594" distance between parallel lines of L1 L9
  measures "d600" distance between parallel lines of L0 L10
  measures "d602" distance from line of point (33, 91.1) L0
  measures "d604" distance from line of point (0, 63.9) L0
  measures "d606" distance from line of point (0, 60.1) L0
  measures "d635" angle of L8 L4
  measures "d636" distance from line of point (33, 91.1) L2
  measures "d637" distance from line of point (0, 63.9) L2
sketch "Sketch29" plane through (0, 2, -91.1) normal (1, 0, 0) x (0, 0, -1)
  line L0 (-16.5, 6) -> (-11.5, 6)
  line L1 (-11.5, 6) -> (-11.5, 8)
  line L2 (-11.5, 8) -> (-16.5, 8)
  line L3 (-16.5, 8) -> (-16.5, 6)
  line L4 (0, 0) -> (-91.1, 0) projected
  line L5 (0, 0) -> (0, 36.2) projected
  point P0 (-91.1, -2)
  point P1 (-28, 0)
  point P2 (-14, 6)
  dimension "d490" = 6
  dimension "d491" = 2
  dimension "d492" = 5
  dimension "d634" = 14
  constraints: 8 end point, 2 parallel, 1 horizontal, 1 midpoint, 1 perpendicular
  measures "d490" distance between parallel lines of L4 L0
  measures "d491" distance between parallel lines of L0 L2
  measures "d492" distance between parallel lines of L3 L1
  measures "d634" distance from line of L5 point (-14, 6)
extrude "Extrusion37" add sketch "Sketch29" along normal blind 2
sketch "Sketch32" plane through (0, 0, 0) normal (0, -1, 0) x (1, 0, 0)
  line L0 (96.1, -63.8) -> (89.1, -63.8) projected
  line L1 (67.6, -46.1) -> (93.6, -46.1)
  line L2 (93.6, -46.1) -> (93.6, -58.8)
  line L3 (93.6, -58.8) -> (67.6, -58.8)
  line L4 (67.6, -58.8) -> (67.6, -46.1)
  line L5 (96.1, 2) -> (96.1, -63.8) projected
  point P0 (0, 0)
  point P1 (73.1, -63.8)
  dimension "d531" = 2.5
  dimension "d532" = 12.7
  dimension "d533" = 26
  dimension "d648" = 5
  constraints: 8 end point, 2 parallel, 1 horizontal, 1 perpendicular
  measures "d531" distance between parallel lines of L5 L2
  measures "d532" distance between parallel lines of L3 L1
  measures "d533" distance between parallel lines of L4 L2
  measures "d648" distance between parallel lines of L0 L3
extrude "Extrusion40" cut sketch "Sketch32" against normal blind 15
sketch "Sketch31" plane through (-2, 0, 2) normal (-1, 0, 0) x (0, 0, 1)
  arc A0 (-10, 26.1471) -> (-13.3807, 27.0529) centre (-11.6904, 26.6) ccw
  line L0 (-14.0192, 11.1471) -> (-10, 26.1471)
  line L1 (-13.0192, 11.1471) -> (-13.5192, 11.1471)
  line L2 (-14.0192, 11.1471) -> (-13.0192, 11.1471)
  line L3 (-17.4, 12.0529) -> (-13.3807, 27.0529)
  arc A1 (-17.4, 12.0529) -> (-14.0192, 11.1471) centre (-15.7096, 11.6) ccw
  line L4 (-95.1, 38.2) -> (0, 38.2)
  arc A2 (-21.2833, 26.1471) -> (-24.6641, 27.0529) centre (-22.9737, 26.6) ccw
  line L5 (-25.3026, 11.1471) -> (-21.2833, 26.1471)
  line L6 (-24.3026, 11.1471) -> (-24.8026, 11.1471)
  line L7 (-25.3026, 11.1471) -> (-24.3026, 11.1471)
  line L8 (-28.6833, 12.0529) -> (-24.6641, 27.0529)
  arc A3 (-28.6833, 12.0529) -> (-25.3026, 11.1471) centre (-26.9929, 11.6) ccw
  arc A4 (-32.5667, 26.1471) -> (-35.9474, 27.0529) centre (-34.257, 26.6) ccw
  line L9 (-36.5859, 11.1471) -> (-32.5667, 26.1471)
  line L10 (-35.5859, 11.1471) -> (-36.0859, 11.1471)
  line L11 (-36.5859, 11.1471) -> (-35.5859, 11.1471)
  line L12 (-39.9667, 12.0529) -> (-35.9474, 27.0529)
  arc A5 (-39.9667, 12.0529) -> (-36.5859, 11.1471) centre (-38.2763, 11.6) ccw
  arc A6 (-43.85, 26.1471) -> (-47.2308, 27.0529) centre (-45.5404, 26.6) ccw
  line L13 (-47.8692, 11.1471) -> (-43.85, 26.1471)
  line L14 (-46.8692, 11.1471) -> (-47.3692, 11.1471)
  line L15 (-47.8692, 11.1471) -> (-46.8692, 11.1471)
  line L16 (-51.25, 12.0529) -> (-47.2308, 27.0529)
  arc A7 (-51.25, 12.0529) -> (-47.8692, 11.1471) centre (-49.5596, 11.6) ccw
  arc A8 (-55.1333, 26.1471) -> (-58.5141, 27.0529) centre (-56.8237, 26.6) ccw
  line L17 (-59.1526, 11.1471) -> (-55.1333, 26.1471)
  line L18 (-58.1526, 11.1471) -> (-58.6526, 11.1471)
  line L19 (-59.1526, 11.1471) -> (-58.1526, 11.1471)
  line L20 (-62.5333, 12.0529) -> (-58.5141, 27.0529)
  arc A9 (-62.5333, 12.0529) -> (-59.1526, 11.1471) centre (-60.843, 11.6) ccw
  arc A10 (-66.4167, 26.1471) -> (-69.7974, 27.0529) centre (-68.1071, 26.6) ccw
  line L21 (-70.4359, 11.1471) -> (-66.4167, 26.1471)
  line L22 (-69.4359, 11.1471) -> (-69.9359, 11.1471)
  line L23 (-70.4359, 11.1471) -> (-69.4359, 11.1471)
  line L24 (-73.8167, 12.0529) -> (-69.7974, 27.0529)
  arc A11 (-73.8167, 12.0529) -> (-70.4359, 11.1471) centre (-72.1263, 11.6) ccw
  arc A12 (-77.7, 26.1471) -> (-81.0808, 27.0529) centre (-79.3904, 26.6) ccw
  line L25 (-81.7193, 11.1471) -> (-77.7, 26.1471)
  line L26 (-80.7193, 11.1471) -> (-81.2193, 11.1471)
  line L27 (-81.7193, 11.1471) -> (-80.7193, 11.1471)
  line L28 (-85.1, 12.0529) -> (-81.0808, 27.0529)
  arc A13 (-85.1, 12.0529) -> (-81.7193, 11.1471) centre (-83.4096, 11.6) ccw
  line L29 (0, 0) -> (0, 38.2) projected
  line L30 (-95.1, 0) -> (-95.1, 38.2) projected
  line L31 (-95.1, 0) -> (0, 0) projected
  line L32 (-95.1, 38.2) -> (0, 38.2) projected
  point P0 (-2, 0)
  point P1 (2, 0)
  point P2 (-15.3904, 19.5529)
  point P3 (-12.0096, 18.6471)
  point P4 (-23.293, 18.6471)
  point P5 (-26.6737, 19.5529)
  point P6 (-34.5763, 18.6471)
  point P7 (-37.957, 19.5529)
  point P8 (-45.8596, 18.6471)
  point P9 (-49.2404, 19.5529)
  point P10 (-57.143, 18.6471)
  point P11 (-60.5237, 19.5529)
  point P12 (-68.4263, 18.6471)
  point P13 (-71.807, 19.5529)
  point P14 (-79.7096, 18.6471)
  point P15 (-83.0904, 19.5529)
  dimension "d509" = 3.5
  dimension "d510" = 15
  dimension "d511" = 75
  dimension "d512" = 1
  dimension "d513" = 11.2833
  dimension "d517" = 10
  dimension "d518" = 10
  dimension "d519" = 11.6
  dimension "d520" = 11.6
  dimension "d522" = 2
  dimension "d523" = 38.2
  constraints: 58 end point, 28 point on circle, 14 centre point, 4 tangent, 3 horizontal, 3 midpoint, 1 parallel, 96 other
  measures "d509" distance between parallel lines of L3 L0
  measures "d510" vertical distance of A1.centre A0.centre
  measures "d511" angle of L0 L2
  measures "d512" distance of L2.start L1.start
  measures "d513" distance of L0.end L5.end
  measures "d517" distance from line of L29 L0.end
  measures "d518" distance from line of L30 L28.start
  measures "d519" distance from line of L31 A1.centre
  measures "d520" distance from line of L32 A0.centre
  measures "d522" distance from line of point (2, 0) L29
  measures "d523" distance from line of point (2, 0) L32
extrude "Extrusion39" cut sketch "Sketch31" against normal blind 15 contours L0 A1 L3 A0 | L5 A3 L8 A2 | L9 A5 L12 A4 | L13 A7 L16 A6 | L17 A9 L20 A8 | L21 A11 L24 A10 | L25 A13 L28 A12
fillet "Fillet1" radius 2 4 edges at (96.1, 19.1, 2) (-2, 19.1, 2) (-2, 19.1, -93.1) (96.1, 15.85, -93.1)
fillet "Fillet3" radius 2 3 edges at (66.1, -3.25, -93.1) (66.1, -3.25, -63.8) (96.1, -3.25, -63.8)
sketch "Sketch34" plane through (96.1, -6.5, -91.1) normal (1, 0, 0) x (0, 0, -1)
  line L0 (-80.872, 17.33) -> (-74.532, 17.33)
  line L1 (-74.532, 14.17) -> (-80.872, 14.17)
  line L2 (-82.172, 16.03) -> (-82.172, 15.47)
  line L3 (-73.232, 16.03) -> (-73.232, 15.47)
  arc A0 (-80.872, 17.33) -> (-82.172, 16.03) centre (-80.872, 16.03) ccw
  arc A1 (-82.172, 15.47) -> (-80.872, 14.17) centre (-80.872, 15.47) ccw
  arc A2 (-74.532, 14.17) -> (-73.232, 15.47) centre (-74.532, 15.47) ccw
  arc A3 (-73.232, 16.03) -> (-74.532, 17.33) centre (-74.532, 16.03) ccw
  line L4 (-93.1, 44.7) -> (-93.1, 6.5) projected
  line L5 (-91.1, 6.5) -> (-25.3, 6.5) projected
  line L6 (-71.202, 20) -> (-84.202, 20)
  line L7 (-84.202, 20) -> (-84.202, 11.5)
  line L8 (-84.202, 11.5) -> (-71.202, 11.5)
  line L9 (-71.202, 11.5) -> (-71.202, 20)
  point P0 (-91.1, 6.5)
  dimension "d551" = 1.3
  dimension "d552" = 6.34
  dimension "d553" = 0.56
  dimension "d554" = 10.928
  dimension "d558" = 5
  dimension "d561" = 8.5
  dimension "d639" = 13
  dimension "d640" = 2.03
  dimension "d641" = 2.03
  dimension "d653" = 2.67
  dimension "d654" = 2.67
  constraints: 16 end point, 8 point on circle, 8 tangent, 4 centre point, 3 equal radius, 2 horizontal, 2 parallel, 2 vertical
  measures "d551" radius of A0
  measures "d552" distance of L0.start L0.end
  measures "d553" distance of L3.start L3.end
  measures "d554" distance between parallel lines of L4 L2
  measures "d558" distance between parallel lines of L5 L8
  measures "d561" distance between parallel lines of L6 L8
  measures "d639" distance of L6.start L6.end
  measures "d640" distance between parallel lines of L9 L3
  measures "d641" distance between parallel lines of L2 L7
  measures "d653" distance between parallel lines of L8 L1
  measures "d654" distance between parallel lines of L6 L0
extrude "Extrusion42" cut sketch "Sketch34" against normal blind 10 contours L0 A3 L3 A2 L1 A1 L2 A0 | L9 L8 L7 L6
sketch "Sketch35" plane through (36, 8, 0) normal (0, 0, -1) x (-1, 0, 0)
  line L0 (-58.1, 30.2) -> (36, 30.2) projected
  line L1 (-40.6, 30.2) -> (-42.1, 30.2)
  line L2 (-42.1, 30.2) -> (-42.1, -6)
  line L3 (-40.6, -6) -> (-40.6, 30.2)
  line L4 (0, -6) -> (3, -6) projected
  circle A0 centre (-38.1, 0.5) radius 2.5 projected
  line L5 (-40.6, -6) -> (-42.1, -6)
  line L6 (-58.1, -6) -> (-58.1, 30.2) projected
  point P0 (36, -8)
  point P1 (33, 31.2)
  point P2 (-40.6, 0.5)
  point P3 (36, 30.2)
  dimension "d564" = 1.5
  dimension "d607" = 16
  constraints: 8 end point, 2 horizontal, 1 horizontal alignment, 1 parallel, 1 perpendicular, 1 point on line, 1 vertical alignment, 3 other
  measures "d564" distance between parallel lines of L3 L2
  measures "d607" distance between parallel lines of L6 L2
extrude "Extrusion43" add sketch "Sketch35" along normal blind 2 contours L0 L3 L5 L2
sketch "Sketch36" plane through (94.1, 36.2, -15) normal (-1, 0, 0) x (0, 0, 1)
  line L0 (-68.1, -29.2) -> (-58.1, -29.2)
  line L1 (-58.1, -29.2) -> (-58.1, -31.2)
  line L2 (-58.1, -31.2) -> (-68.1, -31.2)
  line L3 (-68.1, -31.2) -> (-68.1, -29.2)
  line L4 (15, -36.2) -> (-50.8, -36.2) projected
  line L5 (-78.1, 2) -> (-76.1, 2) projected
  line L6 (-76.1, 2) -> (-76.1, -42.7) projected
  line L7 (-76.1, -42.7) -> (-78.1, -42.7) projected
  line L8 (-78.1, -42.7) -> (-78.1, 2) projected
  point P0 (15, -36.2)
  dimension "d568" = 5
  dimension "d569" = 10
  dimension "d570" = 2
  constraints: 8 end point, 2 parallel, 1 horizontal, 1 perpendicular
  measures "d568" distance between parallel lines of L4 L2
  measures "d569" distance between parallel lines of L3 L1
  measures "d570" distance between parallel lines of L0 L2
extrude "Extrusion44" add sketch "Sketch36" along normal blind 3 contours L0 L1 L2 L3
extrude "Extrusion48" add sketch "Sketch28" along normal blind 6
sketch "Sketch42" plane through (0, 2, 0) normal (0, 1, 0) x (1, 0, 0)
  line L0 (31, 63.1) -> (14, 63.1) projected
  line L1 (14, 63.9) -> (0, 63.9) projected
  line L2 (14, 63.1) -> (14, 63.9) projected
  line L3 (31, 91.1) -> (31, 63.1) projected
  line L4 (0, 63.9) -> (14, 63.9) projected
  line L5 (14, 63.9) -> (14, 63.1) projected
  line L6 (14, 63.1) -> (31, 63.1) projected
  line L7 (31, 63.1) -> (31, 91.1) projected
  line L8 (31, 91.1) -> (0, 91.1) projected
  line L9 (0, 91.1) -> (0, 63.9) projected
  point P0 (0, 0)
extrude "Extrusion53" add sketch "Sketch42" along normal blind 1.5
fillet "Fillet4" radius 0.5 1 edges at (95.1, 13.5, -6.898)
fillet "Fillet5" radius 0.5 3 edges at (95.1, 5, -6.898) (95.1, 13.5, -19.898) (95.1, 5, -19.898)
sketch "Sketch44" plane through (0, 2, 0) normal (0, 1, 0) x (1, 0, 0)
  line L0 (0, 91.1) -> (0, 0) projected
  line L1 (0, 0) -> (10, 0)
  line L2 (10, 0) -> (10, 10)
  line L3 (10, 10) -> (0, 10)
  line L4 (0, 10) -> (0, 0)
  point P0 (0, 19)
  dimension "d649" = 10
  dimension "d650" = 10
  constraints: 8 end point, 2 parallel, 1 horizontal, 1 perpendicular
  measures "d649" distance of L1.end L2.end
  measures "d650" distance of L2.end L3.end
extrude "Extrusion55" cut sketch "Sketch44" against normal blind 10
equation "\"d70\" = d71"
equation "\"d74\" = d75"
equation "\"d81\" = d80"
equation "\"d84\" = d96"
body "Solid1"
